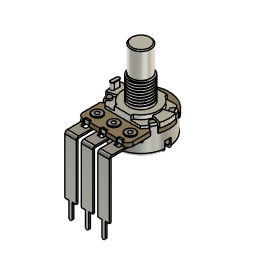
RV16AF-41(LL) (Autodesk Fusion 360 design; units mm, degrees)
Autodesk Fusion 360 part; units mm, degrees
(part 1 of 2)
ref_plane "WorkPlane1" through (0, 0, 1.6) normal (0, 0, 1) x (1, 0, 0)
sketch "Sketch1" plane through (0, 0, 1.6) normal (0, 0, 1) x (1, 0, 0)
  circle A0 centre (0, 0) radius 8.25
  dimension "d2" = 16.5
  constraint coincident A0.centre origin
  measures "d2" diameter of A0
ref_plane "WorkPlane2" through (0, 0, 10.7) normal (0, 0, 1) x (1, 0, 0)
sketch "Sketch2" plane through (0, 0, 10.7) normal (0, 0, 1) x (1, 0, 0)
  line L0 (-10, 5.5) -> (10, 5.5)
  line L1 (-10, -5.5) -> (9.4778, -5.5)
  line L2 (2.5, -5.5) -> (2.5, -4.7864)
  line L3 (2.5, 4.7864) -> (2.5, 5.5)
  line L4 (-2.5, 5.5) -> (-2.5, 4.7864)
  line L5 (-2.5, -4.7864) -> (-2.5, -5.5)
  arc A0 (-2.5, 4.7864) -> (-2.5, -4.7864) centre (0, 0) ccw
  arc A1 (2.5, -4.7864) -> (2.5, 4.7864) centre (0, 0) ccw
  dimension "d4" = 5.5
  dimension "d5" = 5.5
  dimension "d6" = 10.8
  dimension "d7" = 2.5
  dimension "d8" = 2.5
  constraint horizontal L0
  constraint horizontal L1
  constraint coincident A0.centre A1.centre
  constraint perpendicular L0 L2
  constraint perpendicular L1 L4
  constraint coincident L0 L4.start
  constraint coincident L0 L3.end
  constraint coincident L3.start L2
  constraint coincident L2.end A0
  constraint collinear L2 L3
  constraint collinear L4 L5
  constraint coincident L1 L5.end
  constraint coincident L1 L2.start
  constraint concentric A0 A1
  measures "d4" distance of A0.centre L1
  measures "d5" distance of A0.centre L0
  measures "d6" diameter of A0
  measures "d7" distance of A0.centre L2
  measures "d8" distance of A0.centre L4
extrude "Extrude1" add sketch "Sketch2" against normal blind 1.25 makes body 1
sketch "Sketch3" plane through (0, 0, 9.45) normal (0, 0, -1) x (1, 0, 0)
  line L0 (-10, -5.5) -> (5.3531, -5.5)
  line L1 (-5.3531, 5.5) -> (5.3531, 5.5)
  arc A0 (-5.3531, 5.5) -> (-5.3531, -5.5) centre (0, 0) ccw
  arc A1 (5.3531, -5.5) -> (5.3531, 5.5) centre (0, 0) ccw
  dimension "d11" = 5.5
  dimension "d12" = 5.5
  dimension "d13" = 15.35
  constraint horizontal L0
  constraint horizontal L1
  constraint coincident A0.centre A1.centre
  constraint coincident L0.end A0
  constraint coincident L0 A0.end
  constraint concentric A0 A1
  measures "d11" distance of A0.centre L1
  measures "d12" distance of A0.centre L0
  measures "d13" diameter of A0
extrude "Extrude2" add sketch "Sketch3" along normal blind 0.75 bodies 1
ref_plane "WorkPlane3" through (0, 0, 10.2) normal (0, 0, 1) x (1, 0, 0)
sketch "Sketch4" plane through (0, 0, 10.2) normal (0, 0, 1) x (1, 0, 0)
  line L0 (0, 0) -> (-11.5, 0) construction
  line L1 (-8.1393, 2.45) -> (-8.1393, -2.45) construction
  line L2 (-8.1393, 2.45) -> (8.1393, -2.45)
  line L3 (-8.1393, -2.45) -> (8.1393, 2.45)
  arc A0 (-8.1393, 2.45) -> (-8.1393, -2.45) centre (0, 0) ccw
  arc A1 (8.1393, -2.45) -> (8.1393, 2.45) centre (0, 0) ccw
  dimension "d17" = 17
  dimension "d19" = 4.9
  constraint coincident L0.start A0.centre
  constraint perpendicular L0 L1
  constraint horizontal L0
  constraint coincident L2.end A0
  constraint concentric A0 A1
  measures "d17" diameter of A0
  measures "d19" distance of L1.start L1.end
extrude "Extrude3" add sketch "Sketch4" against normal up to surface (1.5 mm away) bodies 1
sketch "Sketch5" plane through (0, 0, 8.7) normal (0, 0, -1) x (1, 0, 0)
  line L0 (0, 0) -> (0, 11.5) construction
  line L1 (0, 10) -> (7.6, 10) construction
  line L2 (7.6, 10) -> (7.6, 3.8066)
  line L3 (-2.5, 5.5) -> (2.5, 5.5) construction
  line L4 (0, 11.5) -> (6.1, 11.5)
  arc A0 (7.6, 10) -> (6.1, 11.5) centre (6.1, 10) ccw
  line L5 (-7.6, 10) -> (-7.6, 3.8066)
  arc A1 (-6.1, 11.5) -> (-7.6, 10) centre (-6.1, 10) ccw
  line L6 (0, 11.5) -> (-6.1, 11.5)
  arc A2 (-7.6, 3.8066) -> (7.6, 3.8066) centre (0, 0) ccw
  circle A3 centre (-5, 8.15) radius 1.55
  circle A4 centre (-5, 8.15) radius 1
  circle A5 centre (0, 8.15) radius 1
  circle A6 centre (0, 8.15) radius 1.55
  circle A7 centre (5, 8.15) radius 1
  circle A8 centre (5, 8.15) radius 1.55
  dimension "d22" = 17
  dimension "d23" = 7.6
  dimension "d24" = 6
  dimension "d25" = 1.5
  dimension "d26" = 3.1
  dimension "d27" = 2
  dimension "d29" = 1.8
  dimension "d30" = 5
  dimension "d31" = 2
  dimension "d32" = 3.1
  dimension "d33" = 2
  dimension "d34" = 3.1
  dimension "d35" = 1.8
  dimension "d36" = 1.8
  dimension "d37" = 5
  constraint coincident L0.start A2.centre
  constraint vertical L0
  constraint coincident L0 L1.start
  constraint perpendicular L0 L1
  constraint perpendicular L1 L2
  constraint perpendicular L0 L4
  constraint coincident L1.end L2
  constraint tangent L4 A0
  constraint tangent L2 A0
  constraint symmetric L4.start L0 L6.start
  constraint symmetric L0 L2.end L5.end
  constraint symmetric L0 L4.end A1.start
  constraint symmetric L0 L1.end L5.start
  constraint symmetric L0 A0 A1
  constraint concentric A3 A4
  constraint coincident L0 A5.centre
  constraint concentric A5 A6
  constraint concentric A7 A8
  measures "d22" diameter of A2
  measures "d23" distance of L1.start L1.end
  measures "d24" distance of L0.end L3
  measures "d25" radius of A0
  measures "d26" diameter of A3
  measures "d27" diameter of A4
  measures "d29" distance of L6 A3
  measures "d30" distance of L0 A3.centre
  measures "d31" diameter of A5
  measures "d32" diameter of A6
  measures "d33" diameter of A7
  measures "d34" diameter of A8
  measures "d35" distance of L6 A6
  measures "d36" distance of L4 A8
  measures "d37" distance of L0 A7.centre
extrude "Extrude4" add sketch "Sketch5" along normal blind 1.24 separate body contours L2 L4 A0 L5 A1 L6 A2 | A3 | A6 | A8 makes body 2
sketch "Sketch6" plane through (0, 0, 7.46) normal (0, 0, -1) x (1, 0, 0)
  circle A0 centre (-5, 8.15) radius 1
  circle A1 centre (0, 8.15) radius 1
  circle A2 centre (5, 8.15) radius 1
  line L0 (-6.74, 8.15) -> (-6.74, 16.25)
  line L1 (-3.26, 8.15) -> (-3.26, 16.25)
  line L2 (-1.74, 8.15) -> (-1.74, 16.25)
  line L3 (1.74, 8.15) -> (1.74, 16.25)
  line L4 (3.26, 8.15) -> (3.26, 16.25)
  line L5 (6.74, 8.15) -> (6.74, 16.25)
  line L6 (0, 0) -> (0, 16.25) construction
  line L7 (0, 16.25) -> (7.5, 16.25) construction
  line L8 (0, 16.25) -> (-7, 16.25) construction
  line L9 (-6.74, 16.25) -> (-3.26, 16.25) construction
  line L10 (-1.74, 16.25) -> (1.74, 16.25) construction
  line L11 (-6.74, 16.25) -> (-3.26, 16.25)
  line L12 (-1.74, 16.25) -> (1.74, 16.25)
  line L13 (3.26, 16.25) -> (6.74, 16.25)
  arc A3 (-6.74, 8.15) -> (-3.26, 8.15) centre (-5, 8.15) ccw
  arc A4 (-1.74, 8.15) -> (1.74, 8.15) centre (0, 8.15) ccw
  arc A5 (3.26, 8.15) -> (6.74, 8.15) centre (5, 8.15) ccw
  dimension "d40" = 3.48
  dimension "d41" = 3.48
  dimension "d42" = 3.48
  dimension "d43" = 16.25
  constraint concentric A0 A3
  constraint concentric A1 A4
  constraint concentric A2 A5
  constraint vertical L0
  constraint parallel L0 L1
  constraint vertical L2
  constraint parallel L1 L3
  constraint vertical L4
  constraint vertical L5
  constraint tangent L5 A5
  constraint tangent L4 A5
  constraint tangent L3 A4
  constraint tangent L2 A4
  constraint tangent L1 A3
  constraint tangent L0 A3
  constraint coincident L6.start origin
  constraint parallel L0 L6
  constraint perpendicular L6 L7
  constraint perpendicular L6 L8
  constraint coincident L7 L3.end
  constraint coincident L7 L4.end
  constraint coincident L7 L5.end
  constraint perpendicular L1 L9
  constraint perpendicular L3 L10
  measures "d40" diameter of A3
  measures "d41" diameter of A4
  measures "d42" diameter of A5
  measures "d43" distance of L6.start L6.end
extrude "Extrude5" add sketch "Sketch6" along normal blind 0.5 separate body makes body 3 at (-5.0249, -13.8824, 7.46) makes body 4 at (-0.0249, -13.8824, 7.46) makes body 5 at (4.9751, -13.8824, 7.46)
sketch "Sketch7" plane through (0, 0, 6.96) normal (0, 0, -1) x (1, 0, 0)
  circle A0 centre (-5, 8.15) radius 1
  line L0 (-6.74, 16.25) -> (-6.74, 8.15)
  arc A1 (-6.74, 8.15) -> (-3.26, 8.15) centre (-5, 8.15) ccw
  line L1 (-3.26, 8.15) -> (-3.26, 16.25)
  line L2 (-3.26, 16.25) -> (-6.74, 16.25)
  circle A2 centre (0, 8.15) radius 1
  line L3 (-1.74, 16.25) -> (-1.74, 8.15)
  arc A3 (-1.74, 8.15) -> (1.74, 8.15) centre (0, 8.15) ccw
  line L4 (1.74, 8.15) -> (1.74, 16.25)
  line L5 (1.74, 16.25) -> (-1.74, 16.25)
  circle A4 centre (5, 8.15) radius 1
  line L6 (3.26, 16.25) -> (3.26, 8.15)
  arc A5 (3.26, 8.15) -> (6.74, 8.15) centre (5, 8.15) ccw
  line L7 (6.74, 8.15) -> (6.74, 16.25)
  line L8 (6.74, 16.25) -> (3.26, 16.25)
  line L9 (-6.74, 15.75) -> (-3.26, 15.75)
  line L10 (-1.74, 15.75) -> (1.74, 15.75)
  line L11 (3.26, 15.75) -> (6.74, 15.75)
  dimension "d46" = 0.5
  constraint coincident L0 L9.start
  constraint perpendicular L0 L9
  constraint coincident L7 L11.end
  constraint coincident L1 L9.end
  constraint coincident L3 L10.start
  constraint collinear L9 L10
  constraint coincident L4 L10.end
  constraint coincident L6 L11.start
  constraint collinear L10 L11
  measures "d46" distance of L2 L9
extrude "Extrude6" add sketch "Sketch7" along normal blind 17.06 contours L0 L1 L2 L9 | L3 L4 L5 L10 | L6 L7 L8 L11 bodies 3 4 5
fillet "Fillet1" radius 0.75 3 edges at (-5, -16.25, 7.46) (0, -16.25, 7.46) (5, -16.25, 7.46) on bodies 3 4 5
fillet "Fillet2" radius 0.25 3 edges at (-5, -15.75, 6.96) (0, -15.75, 6.96) (5, -15.75, 6.96) on bodies 3 4 5
sketch "Sketch9" plane through (0, 0, -10.1) normal (0, 0, -1) x (1, 0, 0)
  line L0 (-6.74, 15.75) -> (-3.26, 15.75)
  line L1 (-3.26, 15.75) -> (-3.26, 16.25)
  line L2 (-3.26, 16.25) -> (-6.74, 16.25)
  line L3 (-6.74, 16.25) -> (-6.74, 15.75)
  line L4 (-1.74, 15.75) -> (1.74, 15.75)
  line L5 (1.74, 15.75) -> (1.74, 16.25)
  line L6 (1.74, 16.25) -> (-1.74, 16.25)
  line L7 (-1.74, 16.25) -> (-1.74, 15.75)
  line L8 (3.26, 15.75) -> (6.74, 15.75)
  line L9 (6.74, 15.75) -> (6.74, 16.25)
  line L10 (6.74, 16.25) -> (3.26, 16.25)
  line L11 (3.26, 16.25) -> (3.26, 15.75)
  line L12 (-5, 16.25) -> (-5, 15.75) construction
  line L13 (-4.5, 16.25) -> (-4.5, 15.75)
  line L14 (-5.5, 16.25) -> (-5.5, 15.75)
  line L15 (0, 16.25) -> (0, 15.75) construction
  line L16 (0.5, 16.25) -> (0.5, 15.75)
  line L17 (-0.5, 16.25) -> (-0.5, 15.75)
  line L18 (5, 16.25) -> (5, 15.75) construction
  line L19 (5.5, 16.25) -> (5.5, 15.75)
  line L20 (4.5, 16.25) -> (4.5, 15.75)
  dimension "d55" = 0.5
  dimension "d56" = 0.5
  dimension "d57" = 0.5
  dimension "d58" = 0.5
  dimension "d59" = 0.5
  dimension "d60" = 0.5
  constraint midpoint L2 L12.start
  constraint midpoint L0 L12.end
  constraint coincident L2 L13.start
  constraint perpendicular L2 L13
  constraint coincident L0 L13.end
  constraint coincident L2 L14.start
  constraint perpendicular L2 L14
  constraint coincident L0 L14.end
  constraint midpoint L6 L15.start
  constraint midpoint L4 L15.end
  constraint coincident L6 L16.start
  constraint coincident L4 L16.end
  constraint perpendicular L4 L16
  constraint coincident L6 L17.start
  constraint perpendicular L6 L17
  constraint coincident L4 L17.end
  constraint midpoint L10 L18.start
  constraint midpoint L8 L18.end
  constraint coincident L10 L19.start
  constraint perpendicular L10 L19
  constraint coincident L8 L19.end
  constraint coincident L10 L20.start
  constraint perpendicular L10 L20
  constraint coincident L8 L20.end
  measures "d55" distance of L15 L16
  measures "d56" distance of L15 L17
  measures "d57" distance of L18 L20
  measures "d58" distance of L18 L19
  measures "d59" distance of L12 L14
  measures "d60" distance of L12 L13
extrude "Extrude7" add sketch "Sketch9" along normal blind 5 contours L0 L2 L13 L14 | L4 L6 L16 L17 | L8 L10 L19 L20 bodies 3 4 5
fillet "Fillet3" radius 0.5 2 edges at (5.5, -16, -15.1) (4.5, -16, -15.1) on bodies 5
fillet "Fillet4" radius 0.5 4 edges at (-5.5, -16, -15.1) (-4.5, -16, -15.1) (-0.5, -16, -15.1) (0.5, -16, -15.1) on bodies 3 4
sketch "Sketch10" plane through (0, 0, 8.7) normal (0, 0, 1) x (-1, 0, 0)
  circle A0 centre (5, 8.15) radius 1
  circle A1 centre (0, 8.15) radius 1
  circle A2 centre (-5, 8.15) radius 1
  circle A3 centre (5, 8.15) radius 1.55
  circle A4 centre (5, 8.15) radius 0.6
  circle A5 centre (0, 8.15) radius 1.55
  circle A6 centre (0, 8.15) radius 0.6
  circle A7 centre (-5, 8.15) radius 0.6
  circle A8 centre (-5, 8.15) radius 1.55
  dimension "d67" = 3.1
  dimension "d68" = 1.2
  dimension "d69" = 3.1
  dimension "d70" = 1.2
  dimension "d71" = 1.2
  dimension "d72" = 3.1
  constraint concentric A0 A3
  constraint concentric A0 A4
  constraint concentric A1 A5
  constraint concentric A1 A6
  constraint concentric A2 A7
  constraint concentric A7 A8
  measures "d67" diameter of A3
  measures "d68" diameter of A4
  measures "d69" diameter of A5
  measures "d70" diameter of A6
  measures "d71" diameter of A7
  measures "d72" diameter of A8
extrude "Extrude8" add sketch "Sketch10" against normal up to surface (1.74 mm away) contours A0 | A1 | A2 bodies 3 4 5
extrude "Extrude9" add sketch "Sketch10" along normal blind 0.26 contours A0 | A1 | A2 | A3 | A5 | A8 bodies 3 4 5
sketch "Sketch11" plane through (0, 0, 7.46) normal (0, 0, -1) x (1, 0, 0)
  circle A0 centre (0, 0) radius 8.25
  dimension "d77" = 16.5
  constraint coincident A0.centre origin
  measures "d77" diameter of A0
extrude "Extrude10" add sketch "Sketch11" along normal blind 5.86 separate body makes body 6
fillet "Fillet5" radius 1 1 edges at (-7.6917, 2.9833, 1.6) on bodies 6
sketch "Sketch12" plane through (0, 0, 7.46) normal (0, 0, 1) x (-1, 0, 0)
  circle A0 centre (0, 0) radius 8.25
  line L0 (0, 0) -> (0, 11) construction
  line L1 (6.15, 5.4991) -> (-6.15, 5.4991)
  dimension "d82" = 12.3
  constraint coincident A0.centre L0.start
  constraint vertical L0
  constraint coincident A0 L1.start
  constraint perpendicular L0 L1
  constraint coincident A0 L1.end
  measures "d82" distance of L1.start L1.end
extrude "Extrude11" cut sketch "Sketch12" against normal blind 2 contours A0 L1 picked at (-0.761, 6.3087) bodies 6
sketch "Sketch13" plane through (0, 0, 8.7) normal (0, 0, 1) x (-1, 0, 0)
  circle A0 centre (0, 0) radius 8.25
  line L0 (-7.6, 10) -> (-7.6, 3.8066) construction
  line L1 (-6.1, 11.5) -> (6.1, 11.5) construction
  line L2 (7.6, 10) -> (7.6, 3.8066) construction
  line L3 (-7.6, 4.67) -> (0, 0)
  line L4 (0, 0) -> (0, 6.5) construction
  line L5 (-7.029, 4.3192) -> (-7.805, 2.6729)
  line L6 (0, 0) -> (-8.0415, 2.7539)
  arc A1 (-7.6, 3.8066) -> (7.6, 3.8066) centre (0, 0) ccw
  line L7 (-7.417, 3.496) -> (-7.0103, 3.3043) construction
  circle A2 centre (0, 0) radius 7.75
  line L8 (0, 0) -> (-10.3, 0) construction
  line L9 (0, 0) -> (-8.0415, -2.7539)
  line L10 (-7.6, -4.67) -> (0, 0)
  line L11 (7.6, -4.67) -> (0, 0)
  line L12 (0, 0) -> (8.0415, -2.7539)
  line L13 (0, 0) -> (8.0415, 2.7539)
  line L14 (7.6, 4.67) -> (0, 0)
  line L15 (-7.6, 3.8066) -> (-7.6, 10)
  line L16 (7.6, 10) -> (7.6, 3.8066)
  dimension "d85" = 16.5
  dimension "d87" = 1.82
  dimension "d174" = 0.5
  constraint coincident A0.centre L3.end
  constraint coincident L0 L3.start
  constraint vertical L4
  constraint symmetric A0.centre L4 L3.end
  constraint coincident L3 L5.start
  constraint coincident A0 L5.start
  constraint coincident A0 L5.end
  constraint coincident A1 L6.end
  constraint coincident L5.end L6
  constraint midpoint L5 L7.start
  constraint perpendicular L5 L7
  constraint concentric A0 A2
  constraint coincident L7.end A2
  constraint perpendicular L4 L8
  constraint symmetric L3.start L8 L10.start
  constraint symmetric A0.centre L8 L3.end
  constraint symmetric L6.end L8 L9.end
  constraint symmetric L3.start L4 L14.start
  constraint symmetric L4 A0.centre L3.end
  constraint symmetric L4 L6.end L13.end
  constraint symmetric L4 L9.end L12.end
  constraint symmetric L4 L10.start L11.start
  measures "d85" diameter of A0
  measures "d87" distance of L5.start L5.end
  measures "d174" distance of A0 A2
extrude "Extrude12" cut sketch "Sketch13" against normal up to surface (1.24 mm away) contours A0 L5 | A0 L3 L6 A1 L15 | L3 L5 L6 A2 | A0 A1 L13 L14 L16 | A0 A2 L13 L14 | A0 A2 L9 L10 | A0 A1 L9 L10 | A0 A2 L11 L12 | A0 A1 L11 L12 bodies 2
extrude "Extrude13" add sketch "Sketch13" against normal up to surface (1.24 mm away) separate body contours A0 L5 | L3 L5 L6 A2 | A0 A2 L13 L14 | A0 A2 L9 L10 | A0 A2 L11 L12 makes body 7 at (7.133, 4.1452, 7.8733) makes body 8 at (7.737, -2.8638, 7.8733) makes body 9 at (-7.737, -2.8638, 8.2867) makes body 10 at (-7.737, 2.8638, 7.8733)
extrude "Extrude14" add 4 faces at (-7.5747, -2.808, 8.7) (-7.5747, 2.808, 8.7) (7.5747, 2.808, 8.7) (7.5747, -2.808, 8.7) along direction (0, 0, 1) up to surface end surface through (0, 0, 9.45) normal (0, 0, 1) offset 0.5 on bodies 7 8 9 10 bodies 9 7 8 10
sketch "Sketch14" plane through (0, 0, 9.95) normal (0, 0, 1) x (-1, 0, 0)
  line L0 (6.603, -4.0574) -> (7.029, -4.3192)
  arc A0 (7.029, -4.3192) -> (7.805, -2.6729) centre (0, 0) ccw
  line L1 (7.805, -2.6729) -> (7.332, -2.5109)
  arc A1 (6.603, -4.0574) -> (7.332, -2.5109) centre (0, 0) ccw
  arc A2 (-7.332, -2.5109) -> (-6.603, -4.0574) centre (0, 0) ccw
  line L2 (-7.332, -2.5109) -> (-7.805, -2.6729)
  arc A3 (-7.805, -2.6729) -> (-7.029, -4.3192) centre (0, 0) ccw
  line L3 (-7.029, -4.3192) -> (-6.603, -4.0574)
  line L4 (-6.603, 4.0574) -> (-7.029, 4.3192)
  arc A4 (-7.029, 4.3192) -> (-7.805, 2.6729) centre (0, 0) ccw
  line L5 (-7.805, 2.6729) -> (-7.332, 2.5109)
  arc A5 (-6.603, 4.0574) -> (-7.332, 2.5109) centre (0, 0) ccw
  arc A6 (7.332, 2.5109) -> (6.603, 4.0574) centre (0, 0) ccw
  line L6 (7.332, 2.5109) -> (7.805, 2.6729)
  arc A7 (7.805, 2.6729) -> (7.029, 4.3192) centre (0, 0) ccw
  line L7 (7.029, 4.3192) -> (6.603, 4.0574)
  circle A8 centre (0, 0) radius 8.25
  line L8 (6.0293, -3.7048) -> (6.603, -4.0574)
  line L9 (7.332, -2.5109) -> (6.6949, -2.2927)
  line L10 (7.332, 2.5109) -> (6.6949, 2.2927)
  line L11 (6.603, 4.0574) -> (6.0293, 3.7048)
  line L12 (-7.332, 2.5109) -> (-6.6949, 2.2927)
  line L13 (-6.603, 4.0574) -> (-6.0293, 3.7048)
  line L14 (-6.603, -4.0574) -> (-6.0293, -3.7048)
  line L15 (-7.332, -2.5109) -> (-6.6949, -2.2927)
  line L16 (5.7626, -2.81) -> (5.8349, -2.6565)
  line L17 (5.8349, 2.6565) -> (5.7626, 2.81)
  line L18 (-5.7626, 2.81) -> (-5.8349, 2.6565)
  line L19 (-5.8349, -2.6565) -> (-5.7626, -2.81)
  arc A9 (5.7626, -2.81) -> (6.0293, -3.7048) centre (6.3958, -3.1084) ccw
  arc A10 (6.6949, -2.2927) -> (5.8349, -2.6565) centre (6.4681, -2.955) ccw
  arc A11 (5.8349, 2.6565) -> (6.6949, 2.2927) centre (6.4681, 2.955) ccw
  arc A12 (6.0293, 3.7048) -> (5.7626, 2.81) centre (6.3958, 3.1084) ccw
  arc A13 (-5.7626, 2.81) -> (-6.0293, 3.7048) centre (-6.3958, 3.1084) ccw
  arc A14 (-6.6949, 2.2927) -> (-5.8349, 2.6565) centre (-6.4681, 2.955) ccw
  arc A15 (-5.8349, -2.6565) -> (-6.6949, -2.2927) centre (-6.4681, -2.955) ccw
  arc A16 (-6.0293, -3.7048) -> (-5.7626, -2.81) centre (-6.3958, -3.1084) ccw
  dimension "d96" = 0.7
  dimension "d97" = 0.7
  dimension "d98" = 0.7
  dimension "d99" = 0.7
  dimension "d100" = 0.7
  dimension "d101" = 0.7
  dimension "d102" = 0.7
  dimension "d103" = 0.7
  constraint concentric A6 A8
  constraint coincident L0.start A1.start
  constraint coincident L1.end A1.end
  constraint coincident A6.start L6.start
  constraint coincident A6.end L7.end
  constraint coincident L5.end A5.end
  constraint coincident L4.start A5.start
  constraint coincident A2.end L3.end
  constraint coincident A2.start L2.start
  constraint parallel L16 L18
  constraint parallel L17 L19
  constraint tangent L8 A9
  constraint tangent L16 A9
  constraint tangent L9 A10
  constraint tangent L16 A10
  constraint tangent L10 A11
  constraint tangent L17 A11
  constraint tangent L11 A12
  constraint tangent L17 A12
  constraint tangent L13 A13
  constraint tangent L18 A13
  constraint tangent L12 A14
  constraint tangent L18 A14
  constraint tangent L15 A15
  constraint tangent L19 A15
  constraint tangent L14 A16
  constraint tangent L19 A16
  measures "d96" radius of A9
  measures "d97" radius of A10
  measures "d98" radius of A11
  measures "d99" radius of A12
  measures "d100" radius of A13
  measures "d101" radius of A14
  measures "d102" radius of A15
  measures "d103" radius of A16
extrude "Extrude15" add sketch "Sketch14" against normal blind 0.5 contours A1 L8 L9 L16 A9 A10 | A2 L14 L15 L19 A15 A16 | A6 L10 L11 L17 A11 A12 | A5 L12 L13 L18 A13 A14 bodies 7 8 9 10
fillet "Fillet6" radius 0.5 4 edges at (7.4626, 3.5175, 9.95) (7.4626, -3.5175, 9.95) (-7.4626, -3.5175, 9.95) (-7.4626, 3.5175, 9.95) on bodies 7 8 9 10
combine "Combine1" operation add target body 6 tool bodies 9 10 7 8
sketch "Sketch15" plane through (0, 0, 10.7) normal (0, 0, 1) x (-1, 0, 0)
  circle A0 centre (0, 0) radius 3.5
  dimension "d108" = 7
  constraint coincident A0.centre origin
  measures "d108" diameter of A0
extrude "Extrude16" add sketch "Sketch15" along normal blind 0.8 bodies 1
sketch "Sketch16" plane through (0, 0, 11.5) normal (0, 0, 1) x (-1, 0, 0)
  circle A0 centre (0, 0) radius 3.5
  dimension "d112" = 7
  constraint coincident A0.centre origin
  measures "d112" diameter of A0
extrude "Extrude17" add sketch "Sketch16" along normal blind 6.2 separate body makes body 11
sketch "Sketch17" plane through (0, 0, 17.7) normal (0, 0, 1) x (-1, 0, 0)
  circle A0 centre (0, 0) radius 3
  dimension "d115" = 6
  constraint coincident A0.centre origin
  measures "d115" diameter of A0
extrude "Extrude18" add sketch "Sketch17" along normal blind 8.2 separate body makes body 12
chamfer "Chamfer2" distance 0.3 angle 45 2 edges at (2.797, 1.0848, 25.9) (2.797, 1.0848, 17.7) on bodies 12
thread "Thread1" "ISO Metric profile 7.0 M7x0.75 6g" major diameter 6.908 minor diameter 6.0475 pitch 0.75 angle 60 modelled right hand crest width 0.1053 on face at (-3.4956, 0.1745, 15.6333) crest through (-3.454, 0, 11.3125) on bodies 11
combine "Combine2" operation add target body 1 tool bodies 11 12
sketch "Sketch19" plane through (0, 0, 10.2) normal (0, 0, 1) x (-1, 0, 0)
  arc A0 (8.1393, -2.45) -> (8.1393, 2.45) centre (0, 0) ccw
  line L0 (0, 0) -> (7.8, 0) construction
  line L1 (7.8, 0) -> (7.8, -1.4) construction
  line L2 (7.8, 0) -> (7.8, 1.4) construction
  line L3 (7.8, 0) -> (8.4, 0) construction
  line L4 (7.8, 0) -> (7.2, 0) construction
  line L5 (8.4, 0.8) -> (8.4, -0.8)
  line L6 (7.2, 0.7997) -> (7.2, -0.8003)
  arc A1 (7.2, -0.7997) -> (8.4, -0.8) centre (7.8, -0.8) ccw
  arc A2 (8.4, 0.8) -> (7.2, 0.7997) centre (7.8, 0.8) ccw
  dimension "d121" = 7.8
  dimension "d122" = 1.4
  dimension "d123" = 1.4
  dimension "d124" = 0.6
  dimension "d125" = 0.6
  constraint coincident A0.centre L0.start
  constraint horizontal L0
  constraint perpendicular L0 L1
  constraint perpendicular L0 L2
  constraint perpendicular L2 L3
  constraint perpendicular L1 L4
  constraint perpendicular L3 L5
  constraint perpendicular L0 L6
  constraint coincident L1.end A1
  constraint coincident L2.end A2
  constraint coincident L3.end L5
  constraint coincident L4.end L6
  constraint coincident L6.end A1
  constraint coincident L6 A1.start
  measures "d121" distance of A0.centre L0.end
  measures "d122" distance of L0.end L1.end
  measures "d123" distance of L0.end L2.end
  measures "d124" distance of L0.end L3.end
  measures "d125" distance of L0.end L4.end
extrude "Extrude20" add sketch "Sketch19" along normal blind 2 bodies 1
fillet "Fillet7" radius 0.1 4 edges at (-7.2, 0, 12.2) (-7.7998, 1.4, 12.2) (-8.4, 0, 12.2) (-7.7998, -1.4, 12.2) on bodies 1
sketch "Sketch20" plane through (0, 0, 7.46) normal (0, 0, 1) x (-1, 0, 0)
  line L0 (-6.1, 11.5) -> (6.1, 11.5)
  line L1 (-6.74, 8.15) -> (-6.74, 15.5)
  line L2 (-3.26, 8.15) -> (-3.26, 15.5)
  line L3 (-1.74, 8.15) -> (-1.74, 15.5)
  line L4 (1.74, 8.15) -> (1.74, 15.5)
  line L5 (3.26, 8.15) -> (3.26, 15.5)
  line L6 (6.74, 8.15) -> (6.74, 15.5)
  line L7 (-4.2, 11.5) -> (-4.2, 11.75)
  line L8 (-4.2, 11.75) -> (-5.8, 11.75)
  line L9 (-5.8, 11.75) -> (-5.8, 11.5)
  line L10 (0.8, 11.5) -> (0.8, 11.75)
  line L11 (-0.8, 11.5) -> (-0.8, 11.75)
  line L12 (0.8, 11.75) -> (-0.8, 11.75)
  line L13 (4.2, 11.5) -> (4.2, 11.75)
  line L14 (4.2, 11.75) -> (5.8, 11.75)
  line L15 (5.8, 11.75) -> (5.8, 11.5)
  line L16 (0.8, 11.5) -> (0.8, 10.75)
  line L17 (0.8, 10.75) -> (-0.8, 10.75)
  line L18 (-0.8, 11.5) -> (-0.8, 10.75)
  line L19 (4.2, 11.5) -> (4.2, 10.75)
  line L20 (4.2, 10.75) -> (5.8, 10.75)
  line L21 (5.8, 10.75) -> (5.8, 11.5)
  line L22 (-4.2, 11.5) -> (-4.2, 10.75)
  line L23 (-4.2, 10.75) -> (-5.8, 10.75)
  line L24 (-5.8, 10.75) -> (-5.8, 11.5)
  dimension "d130" = 0.94
  dimension "d131" = 0.94
  dimension "d132" = 0.25
  dimension "d133" = 0.25
  dimension "d134" = 0.94
  dimension "d135" = 0.94
  dimension "d136" = 0.25
  dimension "d137" = 0.94
  dimension "d138" = 0.94
  dimension "d139" = 0.25
  dimension "d177" = 0.75
  dimension "d178" = 0.75
  dimension "d179" = 0.75
  constraint coincident L0 L7.start
  constraint perpendicular L0 L7
  constraint perpendicular L7 L8
  constraint coincident L0 L9.end
  constraint coincident L0 L10.start
  constraint coincident L0 L11.start
  constraint perpendicular L0 L11
  constraint coincident L0 L13.start
  constraint perpendicular L13 L14
  constraint coincident L0 L15.end
  measures "d130" distance of L2 L7
  measures "d131" distance of L1 L9
  measures "d132" distance of L0 L8
  measures "d133" distance of L10.start L10.end
  measures "d134" distance of L4 L10
  measures "d135" distance of L3 L11
  measures "d136" distance of L11.start L11.end
  measures "d137" distance of L6 L15
  measures "d138" distance of L5 L13
  measures "d139" distance of L13.start L13.end
  measures "d177" distance of L0 L20
  measures "d178" distance of L0 L23
  measures "d179" distance of L0 L17
extrude "Extrude21" cut sketch "Sketch20" along normal up to surface (1.24 mm away) and the other way up to surface (0.5 mm away) bodies 2 3 4 5
fillet "Fillet8" radius 0.1 6 edges at (-5.8, -11.5, 8.08) (-0.8, -11.5, 8.08) (-4.2, -11.5, 8.08) (0.8, -11.5, 8.08) (5.8, -11.5, 8.08) (4.2, -11.5, 8.08) on bodies 2
sketch "Sketch21" plane through (0, -10.75, 0) normal (0, -1, 0) x (1, 0, 0)
  line L0 (-4.2, 7.46) -> (-5.8, 7.46)
  line L1 (-5.8, 7.46) -> (-5.8, 6.96)
  line L2 (-5.8, 6.96) -> (-4.2, 6.96)
  line L3 (-4.2, 6.96) -> (-4.2, 7.46)
  line L4 (0.8, 7.46) -> (-0.8, 7.46)
  line L5 (-0.8, 7.46) -> (-0.8, 6.96)
  line L6 (-0.8, 6.96) -> (0.8, 6.96)
  line L7 (0.8, 6.96) -> (0.8, 7.46)
  line L8 (5.8, 7.46) -> (4.2, 7.46)
  line L9 (4.2, 7.46) -> (4.2, 6.96)
  line L10 (4.2, 6.96) -> (5.8, 6.96)
  line L11 (5.8, 6.96) -> (5.8, 7.46)
  line L12 (-5.8, 7.46) -> (-5.8, 8.7)
  line L13 (-4.2, 7.46) -> (-4.2, 8.7)
  line L14 (-5.8, 8.7) -> (-4.2, 8.7)
  line L15 (-0.8, 7.46) -> (-0.8, 8.7)
  line L16 (0.8, 7.46) -> (0.8, 8.7)
  line L17 (4.2, 7.46) -> (4.2, 8.7)
  line L18 (5.8, 7.46) -> (5.8, 8.7)
  line L19 (5.8, 8.7) -> (4.2, 8.7)
  line L20 (0.8, 8.7) -> (-0.8, 8.7)
  dimension "d146" = 1.24
  dimension "d147" = 1.24
  dimension "d148" = 1.24
  dimension "d149" = 1.24
  dimension "d150" = 1.24
  dimension "d151" = 1.24
  constraint coincident L0.end L1.start
  constraint perpendicular L0 L12
  constraint coincident L0.start L3.end
  constraint perpendicular L0 L13
  constraint coincident L4.end L5.start
  constraint perpendicular L4 L15
  constraint coincident L4.start L7.end
  constraint perpendicular L4 L16
  constraint coincident L8.end L9.start
  constraint perpendicular L8 L17
  constraint coincident L8.start L11.end
  constraint perpendicular L8 L18
  measures "d146" distance of L0.end L12.end
  measures "d147" distance of L0.start L13.end
  measures "d148" distance of L4.end L15.end
  measures "d149" distance of L4.start L16.end
  measures "d150" distance of L8.end L17.end
  measures "d151" distance of L8.start L18.end
extrude "Extrude22" add sketch "Sketch21" along normal blind 0.5 bodies 3 4 5
fillet "Fillet9" radius 0.5 3 edges at (-5, -11.25, 6.96) (0, -11.25, 6.96) (5, -11.25, 6.96) on bodies 3 4 5
extrude "Extrude23" cut 3 faces at (0.2667, -11.75, 7.2933) (-4.7333, -11.75, 7.1267) (4.7333, -11.75, 7.1267) along direction (0, -1, 0) blind 0.74 on bodies 3 4 5 bodies 3 4 5
fillet "Fillet10" radius 0.3 6 edges at (-5.8, -11, 8.7) (-4.2, -11, 8.7) (0.8, -11, 8.7) (-0.8, -11, 8.7) (5.8, -11, 8.7) (4.2, -11, 8.7) on bodies 3 4 5
fillet "Fillet11" radius 0.3 6 edges at (-5.8, -12.49, 7.21) (-4.2, -12.49, 7.21) (0.8, -12.49, 7.21) (-0.8, -12.49, 7.21) (4.2, -12.49, 7.21) (5.8, -12.49, 7.21) on bodies 3 4 5
fillet "Fillet12" radius 0.1 3 edges at (-3.5549, -7.5895, 8.96) (1.4451, -7.5895, 8.96) (6.4451, -7.5895, 8.96) on bodies 3 4 5
sketch "Sketch22" plane through (0, 0, 7.46) normal (0, 0, 1) x (-1, 0, 0)
  line L0 (-7.029, 4.3192) -> (-6.603, 4.0574)
  arc A0 (-6.603, 4.0574) -> (-7.332, 2.5109) centre (0, 0) ccw
  line L1 (-7.332, 2.5109) -> (-7.805, 2.6729)
  arc A1 (-7.805, 2.6729) -> (-7.805, -2.6729) centre (0, 0) ccw
  line L2 (-7.805, -2.6729) -> (-7.332, -2.5109)
  arc A2 (-7.332, -2.5109) -> (-6.603, -4.0574) centre (0, 0) ccw
  line L3 (-6.603, -4.0574) -> (-7.029, -4.3192)
  arc A3 (-7.029, -4.3192) -> (7.029, -4.3192) centre (0, 0) ccw
  line L4 (7.029, -4.3192) -> (6.603, -4.0574)
  arc A4 (6.603, -4.0574) -> (7.332, -2.5109) centre (0, 0) ccw
  line L5 (7.332, -2.5109) -> (7.805, -2.6729)
  arc A5 (7.805, -2.6729) -> (7.805, 2.6729) centre (0, 0) ccw
  line L6 (7.805, 2.6729) -> (7.332, 2.5109)
  arc A6 (7.332, 2.5109) -> (6.603, 4.0574) centre (0, 0) ccw
  line L7 (6.603, 4.0574) -> (7.029, 4.3192)
  arc A7 (7.029, 4.3192) -> (6.15, 5.4991) centre (0, 0) ccw
  line L8 (6.15, 5.4991) -> (-6.15, 5.4991)
  arc A8 (-6.15, 5.4991) -> (-7.029, 4.3192) centre (0, 0) ccw
  circle A9 centre (0, 0) radius 7.75
  dimension "d164" = 0.5
  constraint concentric A0 A9
  measures "d164" distance of A3 A9
extrude "Extrude24" cut sketch "Sketch22" against normal blind 4 contours A0 A2 A4 A6 L8 A9 | L8 A9 bodies 6
split "Split1" by plane through (0, 0, 3.46) normal (0, 0, 1) bodies 6 makes body 13 at (7.4585, -3.5261, 6.1267)
shell "Shell1" thickness 0.5 removed faces 2 at (5.098, -6.0388, 3.46) at (-2.963, -3.0885, 3.46) on bodies 6
combine "Combine3" operation add target body 6 tool bodies 13
sketch "Sketch23" plane through (0, 0, 2.1) normal (0, 0, 1) x (-1, 0, 0)
  spline S0 degree 3 poles (-0.77, -5.3336) (-0.848, -5.3121) (-0.9611, -5.2061) (-1.0921, -5.0315) knots 0 0 0 0 1 1 1 1
  spline S1 degree 3 poles (-1.0921, -5.0315) (-1.271, -4.7933) (-1.3903, -4.5668) (-1.44, -4.3713) knots 0 0 0 0 1 1 1 1
  spline S2 degree 3 poles (-1.44, -4.3713) (-1.4724, -4.2435) (-1.5017, -4.0556) (-1.4984, -3.9962) knots 0 0 0 0 1 1 1 1
  spline S3 degree 3 poles (-1.4984, -3.9962) (-1.494, -3.9184) (-1.4695, -3.8777) (-1.4079, -3.8463) knots 0 0 0 0 1 1 1 1
  spline S4 degree 3 poles (-1.4079, -3.8463) (-1.3653, -3.8245) (-1.3618, -3.824) (-1.2602, -3.8244) knots 0 0 0 0 1 1 1 1
  spline S5 degree 3 poles (-1.2602, -3.8244) (-1.1492, -3.825) (-1.1275, -3.8287) (-0.9585, -3.8768) knots 0 0 0 0 1 1 1 1
  spline S6 degree 3 poles (-0.9585, -3.8768) (-0.8456, -3.9089) (-0.8367, -3.9071) (-0.7835, -3.8413) knots 0 0 0 0 1 1 1 1
  spline S7 degree 3 poles (-0.7835, -3.8413) (-0.7467, -3.7958) (-0.6792, -3.6871) (-0.6792, -3.6733) knots 0 0 0 0 1 1 1 1
  spline S8 degree 3 poles (-0.6792, -3.6733) (-0.6792, -3.6639) (-0.677, -3.6644) (-0.8308, -3.6349) knots 0 0 0 0 1 1 1 1
  spline S9 degree 3 poles (-0.8308, -3.6349) (-1.0364, -3.5953) (-1.308, -3.524) (-1.5038, -3.4581) knots 0 0 0 0 1 1 1 1
  spline S10 degree 3 poles (-1.5038, -3.4581) (-1.6517, -3.4083) (-1.7636, -3.3617) (-1.8995, -3.2935) knots 0 0 0 0 1 1 1 1
  spline S11 degree 3 poles (-1.8995, -3.2935) (-1.9707, -3.2578) (-2.0309, -3.2286) (-2.0333, -3.2286) knots 0 0 0 0 1 1 1 1
  spline S12 degree 3 poles (-2.0333, -3.2286) (-2.0358, -3.2286) (-2.1101, -3.3068) (-2.1984, -3.4024) knots 0 0 0 0 1 1 1 1
  spline S13 degree 3 poles (-2.1984, -3.4024) (-2.815, -4.07) (-3.2644, -4.5162) (-3.339, -4.5349) knots 0 0 0 0 1 1 1 1
  spline S14 degree 3 poles (-3.339, -4.5349) (-3.4155, -4.5541) (-3.6633, -4.2674) (-3.7952, -4.007) knots 0 0 0 0 1 1 1 1
  spline S15 degree 3 poles (-3.7952, -4.007) (-3.8606, -3.8779) (-3.8909, -3.7929) (-3.9336, -3.6182) knots 0 0 0 0 1 1 1 1
  spline S16 degree 3 poles (-3.9336, -3.6182) (-3.9806, -3.4259) (-4, -3.3109) (-4, -3.2238) knots 0 0 0 0 1 1 1 1
  spline S17 degree 3 poles (-4, -3.2238) (-4, -3.1089) (-3.9649, -2.9736) (-3.929, -2.9501) knots 0 0 0 0 1 1 1 1
  spline S18 degree 3 poles (-3.929, -2.9501) (-3.8542, -2.901) (-3.6269, -3.0378) (-3.3934, -3.2724) knots 0 0 0 0 1 1 1 1
  spline S19 degree 3 poles (-3.3934, -3.2724) (-3.3384, -3.3276) (-3.2765, -3.3978) (-3.2559, -3.4283) knots 0 0 0 0 1 1 1 1
  spline S20 degree 3 poles (-3.2559, -3.4283) (-3.228, -3.4696) (-3.2148, -3.4831) (-3.2043, -3.4813) knots 0 0 0 0 1 1 1 1
  spline S21 degree 3 poles (-3.2043, -3.4813) (-3.1835, -3.4778) (-3.1189, -3.412) (-3.061, -3.3356) knots 0 0 0 0 1 1 1 1
  spline S22 degree 3 poles (-3.061, -3.3356) (-2.9423, -3.1787) (-2.7109, -2.8202) (-2.7146, -2.7987) knots 0 0 0 0 1 1 1 1
  spline S23 degree 3 poles (-2.7146, -2.7987) (-2.7158, -2.7918) (-2.7515, -2.7592) (-2.794, -2.7263) knots 0 0 0 0 1 1 1 1
  spline S24 degree 3 poles (-2.794, -2.7263) (-3.0225, -2.5489) (-3.1852, -2.374) (-3.2942, -2.1888) knots 0 0 0 0 1 1 1 1
  spline S25 degree 3 poles (-3.2942, -2.1888) (-3.3716, -2.0573) (-3.408, -1.9578) (-3.4489, -1.7655) knots 0 0 0 0 1 1 1 1
  spline S26 degree 3 poles (-3.4489, -1.7655) (-3.4639, -1.6953) (-3.4954, -1.5671) (-3.5191, -1.4806) knots 0 0 0 0 1 1 1 1
  spline S27 degree 3 poles (-3.5191, -1.4806) (-3.6012, -1.1802) (-3.6212, -1.032) (-3.6376, -0.603) knots 0 0 0 0 1 1 1 1
  spline S28 degree 3 poles (-3.6376, -0.603) (-3.6468, -0.36) (-3.6468, 0.3359) (-3.6375, 0.797) knots 0 0 0 0 1 1 1 1
  line L0 (-3.6375, 0.797) -> (-3.6302, 1.1578)
  line L1 (-3.6302, 1.1578) -> (-3.3077, 1.862)
  spline S29 degree 3 poles (-3.3077, 1.862) (-3.1303, 2.2494) (-2.9775, 2.5746) (-2.9681, 2.5847) knots 0 0 0 0 1 1 1 1
  spline S30 degree 3 poles (-2.9681, 2.5847) (-2.9211, 2.6356) (-2.742, 2.9435) (-2.6971, 3.0507) knots 0 0 0 0 1 1 1 1
  spline S31 degree 3 poles (-2.6971, 3.0507) (-2.6519, 3.1588) (-2.6508, 3.1698) (-2.6726, 3.2969) knots 0 0 0 0 1 1 1 1
  spline S32 degree 3 poles (-2.6726, 3.2969) (-2.6964, 3.4358) (-2.7044, 3.6156) (-2.6913, 3.7193) knots 0 0 0 0 1 1 1 1
  spline S33 degree 3 poles (-2.6913, 3.7193) (-2.6603, 3.9659) (-2.5492, 4.138) (-2.3594, 4.2334) knots 0 0 0 0 1 1 1 1
  spline S34 degree 3 poles (-2.3594, 4.2334) (-2.2374, 4.2947) (-2.1186, 4.3175) (-1.9365, 4.3146) knots 0 0 0 0 1 1 1 1
  line L2 (-1.9365, 4.3146) -> (-1.8144, 4.3127)
  line L3 (-1.8144, 4.3127) -> (-1.2819, 4.5793)
  spline S35 degree 3 poles (-1.2819, 4.5793) (-0.989, 4.726) (-0.7106, 4.8615) (-0.6631, 4.8804) knots 0 0 0 0 1 1 1 1
  spline S36 degree 3 poles (-0.6631, 4.8804) (-0.1973, 5.0665) (0.2313, 5.0357) (0.6497, 4.786) knots 0 0 0 0 1 1 1 1
  spline S37 degree 3 poles (0.6497, 4.786) (0.8294, 4.6787) (1.1561, 4.4186) (1.2079, 4.3416) knots 0 0 0 0 1 1 1 1
  spline S38 degree 3 poles (1.2079, 4.3416) (1.3023, 4.2011) (1.347, 3.8937) (1.3375, 3.4501) knots 0 0 0 0 1 1 1 1
  spline S39 degree 3 poles (1.3375, 3.4501) (1.3215, 2.7113) (1.1602, 1.8491) (0.9314, 1.2793) knots 0 0 0 0 1 1 1 1
  spline S40 degree 3 poles (0.9314, 1.2793) (0.9068, 1.2183) (0.8456, 1.086) (0.7954, 0.9854) knots 0 0 0 0 1 1 1 1
  spline S41 degree 3 poles (0.7954, 0.9854) (0.7451, 0.8847) (0.6853, 0.7586) (0.6625, 0.7051) knots 0 0 0 0 1 1 1 1
  spline S42 degree 3 poles (0.6625, 0.7051) (0.5725, 0.4934) (0.4922, 0.2435) (0.4347, -0.0039) knots 0 0 0 0 1 1 1 1
  spline S43 degree 3 poles (0.4347, -0.0039) (0.3983, -0.1605) (0.3522, -0.4391) (0.3612, -0.4481) knots 0 0 0 0 1 1 1 1
  spline S44 degree 3 poles (0.3612, -0.4481) (0.3656, -0.4525) (0.3918, -0.4471) (0.4325, -0.4334) knots 0 0 0 0 1 1 1 1
  spline S45 degree 3 poles (0.4325, -0.4334) (0.5767, -0.3846) (0.807, -0.333) (0.978, -0.3111) knots 0 0 0 0 1 1 1 1
  spline S46 degree 3 poles (0.978, -0.3111) (1.4358, -0.2526) (1.8279, -0.3456) (2.0944, -0.5759) knots 0 0 0 0 1 1 1 1
  spline S47 degree 3 poles (2.0944, -0.5759) (2.1249, -0.6023) (2.1615, -0.639) (2.1758, -0.6575) knots 0 0 0 0 1 1 1 1
  spline S48 degree 3 poles (2.1758, -0.6575) (2.19, -0.676) (2.2066, -0.6911) (2.2127, -0.691) knots 0 0 0 0 1 1 1 1
  spline S49 degree 3 poles (2.2127, -0.691) (2.2239, -0.6908) (2.2896, -0.6178) (2.8085, -0.0298) knots 0 0 0 0 1 1 1 1
  spline S50 degree 3 poles (2.8085, -0.0298) (3.1138, 0.3163) (3.3107, 0.52) (3.4146, 0.5976) knots 0 0 0 0 1 1 1 1
  spline S51 degree 3 poles (3.4146, 0.5976) (3.6167, 0.7483) (3.7841, 0.773) (3.9989, 0.6836) knots 0 0 0 0 1 1 1 1
  spline S52 degree 3 poles (3.9989, 0.6836) (4.1806, 0.6079) (4.2721, 0.5183) (4.2989, 0.3897) knots 0 0 0 0 1 1 1 1
  spline S53 degree 3 poles (4.2989, 0.3897) (4.3119, 0.3272) (4.3036, 0.2132) (4.2802, 0.1329) knots 0 0 0 0 1 1 1 1
  spline S54 degree 3 poles (4.2802, 0.1329) (4.2371, -0.0149) (4.1932, -0.0886) (3.7686, -0.725) knots 0 0 0 0 1 1 1 1
  spline S55 degree 3 poles (3.7686, -0.725) (3.5098, -1.1128) (3.3644, -1.3243) (3.3537, -1.3284) knots 0 0 0 0 1 1 1 1
  spline S56 degree 3 poles (3.3537, -1.3284) (3.3432, -1.3324) (3.3388, -1.3387) (3.3415, -1.3458) knots 0 0 0 0 1 1 1 1
  spline S57 degree 3 poles (3.3415, -1.3458) (3.3499, -1.3678) (3.4692, -1.4382) (3.6587, -1.5331) knots 0 0 0 0 1 1 1 1
  spline S58 degree 3 poles (3.6587, -1.5331) (3.852, -1.6299) (3.9085, -1.6831) (3.9085, -1.7682) knots 0 0 0 0 1 1 1 1
  spline S59 degree 3 poles (3.9085, -1.7682) (3.9085, -1.821) (3.8792, -1.872) (3.8135, -1.9332) knots 0 0 0 0 1 1 1 1
  spline S60 degree 3 poles (3.8135, -1.9332) (3.756, -1.9868) (3.6412, -2.0586) (3.5367, -2.1063) knots 0 0 0 0 1 1 1 1
  spline S61 degree 3 poles (3.5367, -2.1063) (3.5, -2.1231) (3.4701, -2.1393) (3.4701, -2.1424) knots 0 0 0 0 1 1 1 1
  spline S62 degree 3 poles (3.4701, -2.1424) (3.4701, -2.1455) (3.4844, -2.1579) (3.5019, -2.1699) knots 0 0 0 0 1 1 1 1
  spline S63 degree 3 poles (3.5019, -2.1699) (3.5519, -2.2044) (3.6218, -2.2839) (3.6469, -2.335) knots 0 0 0 0 1 1 1 1
  spline S64 degree 3 poles (3.6469, -2.335) (3.6944, -2.4316) (3.7019, -2.5371) (3.6702, -2.6612) knots 0 0 0 0 1 1 1 1
  spline S65 degree 3 poles (3.6702, -2.6612) (3.6248, -2.8385) (3.5218, -2.9231) (3.3076, -2.9589) knots 0 0 0 0 1 1 1 1
  spline S66 degree 3 poles (3.3076, -2.9589) (3.2451, -2.9694) (3.2052, -2.971) (3.097, -2.9674) knots 0 0 0 0 1 1 1 1
  spline S67 degree 3 poles (3.097, -2.9674) (2.9532, -2.9625) (2.8717, -2.9519) (2.7165, -2.9178) knots 0 0 0 0 1 1 1 1
  spline S68 degree 3 poles (2.7165, -2.9178) (2.6621, -2.9059) (2.6147, -2.8979) (2.6112, -2.9) knots 0 0 0 0 1 1 1 1
  spline S69 degree 3 poles (2.6112, -2.9) (2.6078, -2.9021) (2.5909, -2.9275) (2.5737, -2.9564) knots 0 0 0 0 1 1 1 1
  spline S70 degree 3 poles (2.5737, -2.9564) (2.5395, -3.0141) (2.4545, -3.0938) (2.2053, -3.302) knots 0 0 0 0 1 1 1 1
  spline S71 degree 3 poles (2.2053, -3.302) (1.8737, -3.5791) (1.6452, -3.7328) (1.5064, -3.7721) knots 0 0 0 0 1 1 1 1
  spline S72 degree 3 poles (1.5064, -3.7721) (1.482, -3.779) (1.4138, -3.8075) (1.3548, -3.8355) knots 0 0 0 0 1 1 1 1
  spline S73 degree 3 poles (1.3548, -3.8355) (1.1997, -3.909) (1.1075, -3.9254) (0.9369, -3.9097) knots 0 0 0 0 1 1 1 1
  spline S74 degree 3 poles (0.9369, -3.9097) (0.7826, -3.8954) (0.5059, -3.838) (0.2935, -3.7762) knots 0 0 0 0 1 1 1 1
  spline S75 degree 3 poles (0.2935, -3.7762) (0.265, -3.7679) (0.2348, -3.7611) (0.2263, -3.7611) knots 0 0 0 0 1 1 1 1
  spline S76 degree 3 poles (0.2263, -3.7611) (0.2043, -3.7611) (0.1649, -3.8441) (-0.0158, -4.2714) knots 0 0 0 0 1 1 1 1
  spline S77 degree 3 poles (-0.0158, -4.2714) (-0.1832, -4.667) (-0.2805, -4.8687) (-0.3645, -4.994) knots 0 0 0 0 1 1 1 1
  spline S78 degree 3 poles (-0.3645, -4.994) (-0.4121, -5.0651) (-0.5735, -5.2598) (-0.6078, -5.2876) knots 0 0 0 0 1 1 1 1
  spline S79 degree 3 poles (-0.6078, -5.2876) (-0.6687, -5.3369) (-0.7126, -5.3494) (-0.7699, -5.3336) knots 0 0 0 0 1 1 1 1
  line L4 (-0.7699, -5.3336) -> (-0.77, -5.3336)
  spline S80 degree 3 poles (-0.6357, -4.9895) (-0.4981, -4.8915) (-0.2879, -4.446) (-0.073, -3.7971) knots 0 0 0 0 1 1 1 1
  spline S81 degree 3 poles (-0.073, -3.7971) (-0.021, -3.64) (-0.0095, -3.6002) (-0.0066, -3.5666) knots 0 0 0 0 1 1 1 1
  spline S82 degree 3 poles (-0.0066, -3.5666) (-0.0063, -3.5633) (0.0052, -3.5559) (0.019, -3.5502) knots 0 0 0 0 1 1 1 1
  spline S83 degree 3 poles (0.019, -3.5502) (0.095, -3.5184) (0.3079, -3.5327) (0.7335, -3.5983) knots 0 0 0 0 1 1 1 1
  spline S84 degree 3 poles (0.7335, -3.5983) (1.0222, -3.6427) (1.1397, -3.6435) (1.2854, -3.6019) knots 0 0 0 0 1 1 1 1
  spline S85 degree 3 poles (1.2854, -3.6019) (1.4729, -3.5484) (1.7349, -3.3734) (2.1808, -3.0036) knots 0 0 0 0 1 1 1 1
  spline S86 degree 3 poles (2.1808, -3.0036) (2.2801, -2.9213) (2.324, -2.8803) (2.327, -2.8668) knots 0 0 0 0 1 1 1 1
  spline S87 degree 3 poles (2.327, -2.8668) (2.3294, -2.8563) (2.3464, -2.8177) (2.3647, -2.7811) knots 0 0 0 0 1 1 1 1
  spline S88 degree 3 poles (2.3647, -2.7811) (2.4039, -2.703) (2.418, -2.6424) (2.4243, -2.526) knots 0 0 0 0 1 1 1 1
  spline S89 degree 3 poles (2.4243, -2.526) (2.4337, -2.3506) (2.3925, -2.1465) (2.313, -1.9744) knots 0 0 0 0 1 1 1 1
  spline S90 degree 3 poles (2.313, -1.9744) (2.2503, -1.8387) (2.1244, -1.6833) (2.0047, -1.5941) knots 0 0 0 0 1 1 1 1
  spline S91 degree 3 poles (2.0047, -1.5941) (1.7648, -1.4152) (1.4192, -1.3436) (0.899, -1.3652) knots 0 0 0 0 1 1 1 1
  spline S92 degree 3 poles (0.899, -1.3652) (0.6873, -1.374) (0.6828, -1.3739) (0.6318, -1.3584) knots 0 0 0 0 1 1 1 1
  spline S93 degree 3 poles (0.6318, -1.3584) (0.55, -1.3336) (0.4675, -1.2491) (0.4976, -1.221) knots 0 0 0 0 1 1 1 1
  spline S94 degree 3 poles (0.4976, -1.221) (0.5247, -1.1954) (0.7434, -1.1242) (0.9044, -1.0884) knots 0 0 0 0 1 1 1 1
  spline S95 degree 3 poles (0.9044, -1.0884) (1.0664, -1.0524) (1.153, -1.0435) (1.3437, -1.0435) knots 0 0 0 0 1 1 1 1
  spline S96 degree 3 poles (1.3437, -1.0435) (1.5308, -1.0434) (1.6318, -1.0551) (1.7584, -1.0913) knots 0 0 0 0 1 1 1 1
  spline S97 degree 3 poles (1.7584, -1.0913) (1.8046, -1.1045) (1.8103, -1.1047) (1.8265, -1.0941) knots 0 0 0 0 1 1 1 1
  spline S98 degree 3 poles (1.8265, -1.0941) (1.8543, -1.0759) (2.0206, -0.9108) (2.0205, -0.9016) knots 0 0 0 0 1 1 1 1
  spline S99 degree 3 poles (2.0205, -0.9016) (2.0203, -0.8832) (1.8693, -0.7828) (1.7554, -0.7252) knots 0 0 0 0 1 1 1 1
  spline S100 degree 3 poles (1.7554, -0.7252) (1.6223, -0.658) (1.4598, -0.6055) (1.3152, -0.5831) knots 0 0 0 0 1 1 1 1
  spline S101 degree 3 poles (1.3152, -0.5831) (1.2038, -0.5657) (0.9647, -0.5659) (0.837, -0.5834) knots 0 0 0 0 1 1 1 1
  spline S102 degree 3 poles (0.837, -0.5834) (0.6327, -0.6114) (0.3431, -0.6955) (0.3302, -0.7306) knots 0 0 0 0 1 1 1 1
  spline S103 degree 3 poles (0.3302, -0.7306) (0.3284, -0.7356) (0.3243, -0.7814) (0.3212, -0.8322) knots 0 0 0 0 1 1 1 1
  line L5 (0.3212, -0.8322) -> (0.3156, -0.9247)
  line L6 (0.3156, -0.9247) -> (0.2424, -0.923)
  spline S104 degree 3 poles (0.2424, -0.923) (0.1602, -0.9211) (0.0836, -0.9047) (0.0696, -0.886) knots 0 0 0 0 1 1 1 1
  spline S105 degree 3 poles (0.0696, -0.886) (0.046, -0.8546) (0.0431, -0.8181) (0.0401, -0.5274) knots 0 0 0 0 1 1 1 1
  spline S106 degree 3 poles (0.0401, -0.5274) (0.0376, -0.2733) (0.0389, -0.2253) (0.0497, -0.1723) knots 0 0 0 0 1 1 1 1
  spline S107 degree 3 poles (0.0497, -0.1723) (0.0665, -0.0894) (0.1267, 0.1054) (0.2126, 0.3548) knots 0 0 0 0 1 1 1 1
  spline S108 degree 3 poles (0.2126, 0.3548) (0.551, 1.3374) (0.7515, 1.9901) (0.91, 2.6254) knots 0 0 0 0 1 1 1 1
  spline S109 degree 3 poles (0.91, 2.6254) (0.9946, 2.9647) (1.0213, 3.1229) (1.0271, 3.3207) knots 0 0 0 0 1 1 1 1
  spline S110 degree 3 poles (1.0271, 3.3207) (1.0363, 3.6323) (0.9813, 3.8052) (0.7504, 4.1909) knots 0 0 0 0 1 1 1 1
  spline S111 degree 3 poles (0.7504, 4.1909) (0.6297, 4.3925) (0.5653, 4.4717) (0.4532, 4.5566) knots 0 0 0 0 1 1 1 1
  spline S112 degree 3 poles (0.4532, 4.5566) (0.3673, 4.6216) (0.2611, 4.6728) (0.1524, 4.7015) knots 0 0 0 0 1 1 1 1
  spline S113 degree 3 poles (0.1524, 4.7015) (0.0678, 4.7239) (0.0581, 4.7248) (-0.0838, 4.7251) knots 0 0 0 0 1 1 1 1
  spline S114 degree 3 poles (-0.0838, 4.7251) (-0.2414, 4.7254) (-0.2964, 4.7183) (-0.4275, 4.6803) knots 0 0 0 0 1 1 1 1
  spline S115 degree 3 poles (-0.4275, 4.6803) (-0.5045, 4.658) (-1.1223, 4.3947) (-1.1645, 4.3662) knots 0 0 0 0 1 1 1 1
  spline S116 degree 3 poles (-1.1645, 4.3662) (-1.1813, 4.3548) (-1.2429, 4.322) (-1.3014, 4.2931) knots 0 0 0 0 1 1 1 1
  spline S117 degree 3 poles (-1.3014, 4.2931) (-1.3598, 4.2642) (-1.4105, 4.2378) (-1.414, 4.2343) knots 0 0 0 0 1 1 1 1
  spline S118 degree 3 poles (-1.414, 4.2343) (-1.4175, 4.2308) (-1.402, 4.1956) (-1.3792, 4.1552) knots 0 0 0 0 1 1 1 1
  spline S119 degree 3 poles (-1.3792, 4.1552) (-1.2279, 3.8874) (-1.1741, 3.6981) (-1.1993, 3.5222) knots 0 0 0 0 1 1 1 1
  spline S120 degree 3 poles (-1.1993, 3.5222) (-1.2041, 3.4883) (-1.2033, 3.4797) (-1.1953, 3.4797) knots 0 0 0 0 1 1 1 1
  spline S121 degree 3 poles (-1.1953, 3.4797) (-1.1898, 3.4797) (-1.1409, 3.4992) (-1.0867, 3.5232) knots 0 0 0 0 1 1 1 1
  spline S122 degree 3 poles (-1.0867, 3.5232) (-1.0317, 3.5475) (-0.982, 3.565) (-0.9742, 3.563) knots 0 0 0 0 1 1 1 1
  spline S123 degree 3 poles (-0.9742, 3.563) (-0.9489, 3.5564) (-0.9022, 3.504) (-0.8938, 3.4729) knots 0 0 0 0 1 1 1 1
  spline S124 degree 3 poles (-0.8938, 3.4729) (-0.8851, 3.4404) (-0.8889, 3.4156) (-0.9088, 3.3761) knots 0 0 0 0 1 1 1 1
  spline S125 degree 3 poles (-0.9088, 3.3761) (-0.9298, 3.3345) (-0.9584, 3.3139) (-1.0527, 3.2727) knots 0 0 0 0 1 1 1 1
  spline S126 degree 3 poles (-1.0527, 3.2727) (-1.1881, 3.2135) (-1.4071, 3.1006) (-1.4833, 3.0506) knots 0 0 0 0 1 1 1 1
  spline S127 degree 3 poles (-1.4833, 3.0506) (-1.5908, 2.9801) (-1.6134, 2.9354) (-1.5573, 2.9048) knots 0 0 0 0 1 1 1 1
  spline S128 degree 3 poles (-1.5573, 2.9048) (-1.5372, 2.8937) (-1.5154, 2.8918) (-1.4188, 2.8924) knots 0 0 0 0 1 1 1 1
  spline S129 degree 3 poles (-1.4188, 2.8924) (-1.2856, 2.8932) (-1.2603, 2.8996) (-1.2661, 2.9305) knots 0 0 0 0 1 1 1 1
  spline S130 degree 3 poles (-1.2661, 2.9305) (-1.2785, 2.9967) (-1.2788, 3.0342) (-1.267, 3.0461) knots 0 0 0 0 1 1 1 1
  spline S131 degree 3 poles (-1.267, 3.0461) (-1.2331, 3.08) (-1.1553, 3.0458) (-1.0683, 2.9589) knots 0 0 0 0 1 1 1 1
  spline S132 degree 3 poles (-1.0683, 2.9589) (-1.0108, 2.9013) (-0.9842, 2.8522) (-0.9925, 2.819) knots 0 0 0 0 1 1 1 1
  spline S133 degree 3 poles (-0.9925, 2.819) (-1.0046, 2.7709) (-1.0726, 2.7346) (-1.1919, 2.7126) knots 0 0 0 0 1 1 1 1
  spline S134 degree 3 poles (-1.1919, 2.7126) (-1.3247, 2.688) (-1.6981, 2.6983) (-1.8213, 2.7299) knots 0 0 0 0 1 1 1 1
  spline S135 degree 3 poles (-1.8213, 2.7299) (-1.9062, 2.7517) (-1.9733, 2.7999) (-1.9853, 2.8477) knots 0 0 0 0 1 1 1 1
  spline S136 degree 3 poles (-1.9853, 2.8477) (-1.9964, 2.8918) (-1.9843, 2.9537) (-1.9526, 3.0146) knots 0 0 0 0 1 1 1 1
  spline S137 degree 3 poles (-1.9526, 3.0146) (-1.9356, 3.0473) (-1.9217, 3.0755) (-1.9217, 3.0772) knots 0 0 0 0 1 1 1 1
  spline S138 degree 3 poles (-1.9217, 3.0772) (-1.9217, 3.0789) (-1.9525, 3.0803) (-1.9901, 3.0803) knots 0 0 0 0 1 1 1 1
  spline S139 degree 3 poles (-1.9901, 3.0803) (-2.0753, 3.0804) (-2.1738, 3.095) (-2.2986, 3.126) knots 0 0 0 0 1 1 1 1
  spline S140 degree 3 poles (-2.2986, 3.126) (-2.3592, 3.1411) (-2.3973, 3.1473) (-2.4015, 3.1428) knots 0 0 0 0 1 1 1 1
  spline S141 degree 3 poles (-2.4015, 3.1428) (-2.4085, 3.1353) (-2.543, 2.7343) (-2.543, 2.7211) knots 0 0 0 0 1 1 1 1
  spline S142 degree 3 poles (-2.543, 2.7211) (-2.543, 2.7167) (-2.5126, 2.7091) (-2.4746, 2.704) knots 0 0 0 0 1 1 1 1
  spline S143 degree 3 poles (-2.4746, 2.704) (-2.2448, 2.6734) (-1.4433, 2.4959) (-0.8641, 2.3472) knots 0 0 0 0 1 1 1 1
  spline S144 degree 3 poles (-0.8641, 2.3472) (-0.2563, 2.1912) (0.0822, 2.0862) (0.1185, 2.0424) knots 0 0 0 0 1 1 1 1
  spline S145 degree 3 poles (0.1185, 2.0424) (0.1259, 2.0335) (0.124, 2.0287) (0.1081, 2.0162) knots 0 0 0 0 1 1 1 1
  spline S146 degree 3 poles (0.1081, 2.0162) (0.0973, 2.0078) (0.0764, 1.9983) (0.0616, 1.9951) knots 0 0 0 0 1 1 1 1
  spline S147 degree 3 poles (0.0616, 1.9951) (0.024, 1.9871) (-0.1297, 1.9895) (-0.2095, 1.9994) knots 0 0 0 0 1 1 1 1
  spline S148 degree 3 poles (-0.2095, 1.9994) (-0.2461, 2.0039) (-0.3159, 2.011) (-0.3645, 2.0153) knots 0 0 0 0 1 1 1 1
  spline S149 degree 3 poles (-0.3645, 2.0153) (-0.4668, 2.0242) (-0.6742, 2.0583) (-1.1329, 2.1415) knots 0 0 0 0 1 1 1 1
  spline S150 degree 3 poles (-1.1329, 2.1415) (-1.5012, 2.2084) (-2.2365, 2.3462) (-2.4986, 2.3974) knots 0 0 0 0 1 1 1 1
  spline S151 degree 3 poles (-2.4986, 2.3974) (-2.5942, 2.4161) (-2.6806, 2.4318) (-2.6907, 2.4323) knots 0 0 0 0 1 1 1 1
  spline S152 degree 3 poles (-2.6907, 2.4323) (-2.708, 2.4331) (-2.7244, 2.3977) (-2.9996, 1.7649) knots 0 0 0 0 1 1 1 1
  line L7 (-2.9996, 1.7649) -> (-3.2903, 1.0967)
  line L8 (-3.2903, 1.0967) -> (-3.3085, 0.9846)
  spline S153 degree 3 poles (-3.3085, 0.9846) (-3.3959, 0.4464) (-3.4187, -0.2206) (-3.3673, -0.7361) knots 0 0 0 0 1 1 1 1
  spline S154 degree 3 poles (-3.3673, -0.7361) (-3.2936, -1.4736) (-3.0683, -2.0514) (-2.71, -2.4215) knots 0 0 0 0 1 1 1 1
  spline S155 degree 3 poles (-2.71, -2.4215) (-2.6224, -2.512) (-2.5398, -2.5808) (-2.409, -2.6721) knots 0 0 0 0 1 1 1 1